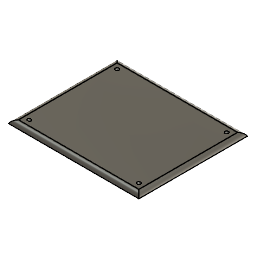
Electronics_Enclosure_Lid (Autodesk Fusion 360 design; units mm, degrees)
Autodesk Fusion 360 part; units mm, degrees
sketch "Sketch1" plane through (0, 0, 0) normal (0, 0, 1) x (1, 0, 0)
  line L0 (0, 0) -> (120, 0)
  line L1 (120, 0) -> (120, 100)
  line L2 (120, 100) -> (0, 100)
  line L3 (0, 100) -> (0, 0)
  dimension "d1" = 100
  dimension "d2" = 120
  constraint horizontal L0
  constraint vertical L1
  constraint horizontal L2
  constraint vertical L3
  constraint coincident L0.start L3.end
  measures "d1" distance of L0.start L2.end
  measures "d2" distance of L0.start L0.end
extrude "Extrude1" add sketch "Sketch1" along normal blind 3
fillet "Fillet1" radius 5 4 edges at (0, 50, 3) (60, 0, 3) (120, 50, 3) (60, 100, 3)
sketch "Sketch2" plane through (0, 0, 3) normal (0, 0, 1) x (-1, 0, 0)
  line L0 (-115.4174, -4.5826) -> (-115.4174, -95.4174)
  line L1 (-115.4174, -95.4174) -> (-4.5826, -95.4174)
  line L2 (-4.5826, -95.4174) -> (-4.5826, -4.5826)
  line L3 (-4.5826, -4.5826) -> (-115.4174, -4.5826)
  circle A0 centre (-9.5826, -90.4174) radius 1.6
  circle A1 centre (-110.4174, -90.4174) radius 1.6
  circle A2 centre (-9.5826, -9.5826) radius 1.6
  circle A3 centre (-110.4174, -9.5826) radius 1.6
  dimension "d7" = 3.2
  dimension "d8" = 3.2
  dimension "d9" = 3.2
  dimension "d10" = 3.2
  dimension "d11" = 5
  dimension "d12" = 5
  dimension "d13" = 5
  dimension "d14" = 5
  dimension "d15" = 5
  dimension "d16" = 5
  dimension "d17" = 5
  dimension "d18" = 5
  measures "d7" diameter of A0
  measures "d8" diameter of A1
  measures "d9" diameter of A2
  measures "d10" diameter of A3
  measures "d11" distance of L2 A2.centre
  measures "d12" distance of L3 A2.centre
  measures "d13" distance of L3 A3.centre
  measures "d14" distance of L0 A3.centre
  measures "d15" distance of L1 A0.centre
  measures "d16" distance of L2 A0.centre
  measures "d17" distance of L0 A1.centre
  measures "d18" distance of L1 A1.centre
extrude "Extrude2" cut sketch "Sketch2" against normal blind 10 contours A0 | A1 | A2 | A3
